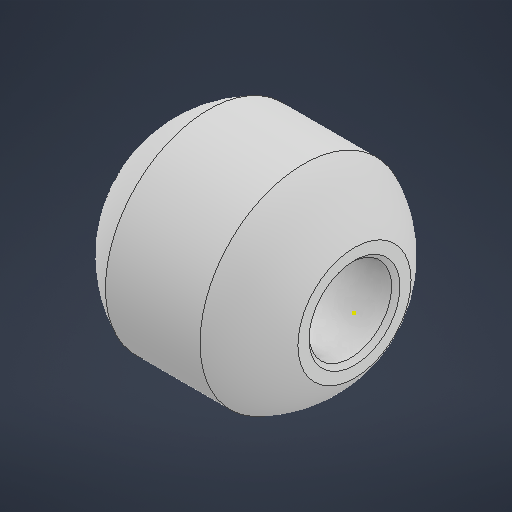
# Autodesk Inventor part: mắt trâu
Saved by Autodesk Inventor 2027.1 (Build 311270010, 270A)
## iProperties
Created: 2026-08-09
Part Number: mắt trâu
Material: Generic
Document SubType Name: Sheet Metal
Designer: MSI
Density: 1 g/cm^3
Sheet Metal Rule: Default_mm
Appearance: Default
Author: MSI
Autodesk Inventor part; units mm, degrees
ref_plane "YZ Plane" through (0, 0, 0) normal (1, 0, 0) x (0, 1, 0)
ref_plane "XZ Plane" through (0, 0, 0) normal (0, 1, 0) x (-1, 0, 0)
ref_plane "XY Plane" through (0, 0, 0) normal (0, 0, 1) x (1, 0, 0)
sketch "Sketch1" plane through (0, 0, 0) normal (0, 0, 1) x (1, 0, 0)
  line L0 (-4.7685, 2) -> (4.7685, 2)
  line L1 (4.7685, 2) -> (4.7685, 2.7408)
  line L2 (-4.7685, 2) -> (-4.7685, 2.7408)
  line L3 (0, 0) -> (2.529, 0)
  arc A0 (4.7685, 2.7408) -> (-4.7685, 2.7408) centre (0, 0) ccw
  dimension "d1" = 2
  dimension "d8" = 11
  constraints: 8 end point, 2 horizontal, 2 point on circle, 1 centre point, 1 coincident, 1 vertical
  measures "d1" distance from line of point (0, 0) L0
  measures "d8" diameter of A0
revolve "Revolution1" add sketch "Sketch1" angle 360 about axis through (0, 0, 0) along (1, 0, 0)
sketch "Sketch2" plane through (4.7685, 0, 0) normal (1, 0, 0) x (0, 0, -1)
  circle A0 centre (0, 0) radius 6
  circle A1 centre (0, 0) radius 2 projected
  circle A2 centre (0, 0) radius 5
  dimension "d5" = 10
  constraints: 2 centre point, 2 coincident
  measures "d5" diameter of A2
extrude "Extrusion1" cut sketch "Sketch2" against normal blind 10 contours A0
sketch "Sketch3" plane through (4.7685, 0, 0) normal (1, 0, 0) x (0, 0, -1)
  point P0 (0, 0)
sketch "Sketch4" plane through (4.7685, 0, 0) normal (1, 0, 0) x (0, 0, -1)
  point P0 (0, 0)
chamfer "Chamfer1" distance 0.2 angle 45 2 edges at (4.7685, -2, 0) (-4.7685, -2, 0)
equation "\"BendRadius\" = Thickness"
equation "\"BendReliefWidth\" = Thickness"
equation "\"BendReliefDepth\" = 0.5 * Thickness"
equation "\"CornerReliefSize\" = 4 * Thickness"
equation "\"MinimumRemnant\" = 2 * Thickness"
equation "\"TransitionRadius\" = BendRadius"
equation "\"JacobiRadiusSize\" = BendRadius"
equation "\"GapSize\" = Thickness"
equation "\"Thickness\" = 0.5"
body "Solid1"
